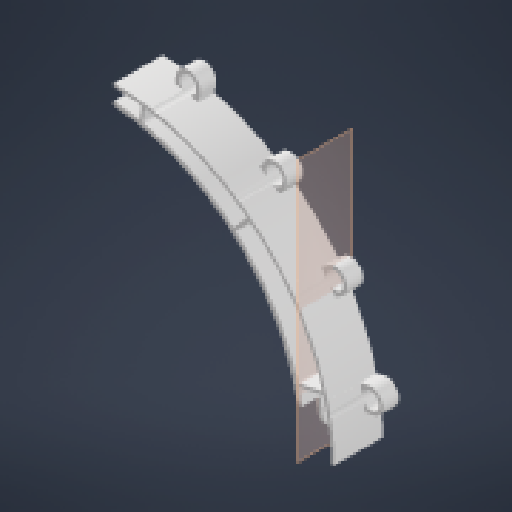
# Autodesk Inventor part: FilterSidewall
Saved by Autodesk Inventor 2026 (Build 300175050, 175E)
## iProperties
Created: 2026-05-05
Part Number: FilterSidewall
Material: Generic
Document SubType Name: Modeling
Designer: sniel
Density: 1 g/cm^3
Appearance: Default
Author: sniel
Autodesk Inventor part; units mm, degrees
ref_plane "YZ Plane" through (0, 0, 0) normal (1, 0, 0) x (0, 1, 0)
ref_plane "XZ Plane" through (0, 0, 0) normal (0, 1, 0) x (-1, 0, 0)
ref_plane "XY Plane" through (0, 0, 0) normal (0, 0, 1) x (1, 0, 0)
sketch "Sketch1" plane through (0, 0, 0) normal (0, 0, 1) x (1, 0, 0)
  circle A0 centre (-26.4627, 2.4988) radius 5.25
  circle A1 centre (-79.388, -19.4236) radius 5.25
  circle A2 centre (-138.7343, -109.7729) radius 5.25
  circle A3 centre (-116.8119, -56.8475) radius 5.25
  line L0 (-70.3746, -19.4683) -> (-73.0753, -15.2583)
  arc A4 (-73.0753, -15.2583) -> (-85.477, -23.6867) centre (-79.3881, -19.3078) ccw
  line L1 (-85.477, -23.6867) -> (-82.5566, -27.7475)
  arc A5 (-82.5566, -27.7475) -> (-108.3722, -53.5631) centre (0, -136.1197) ccw
  line L2 (-108.3722, -53.5631) -> (-112.433, -50.6428)
  arc A6 (-112.433, -50.6428) -> (-120.8615, -63.0445) centre (-116.8119, -56.7317) ccw
  line L3 (-120.8615, -63.0445) -> (-116.6514, -65.7451)
  arc A7 (-116.6514, -65.7451) -> (-132.2473, -103.397) centre (0, -136.1197) ccw
  line L4 (-132.2473, -103.397) -> (-137.134, -102.3297)
  arc A8 (-137.134, -102.3297) -> (-139.9435, -117.0589) centre (-138.7343, -109.657) ccw
  line L5 (-139.9435, -117.0589) -> (-135.0071, -117.8653)
  arc A9 (-135.0071, -117.8653) -> (-136.2355, -136.2355) centre (0, -136.1197) ccw
  line L6 (-136.2355, -136.2355) -> (-134.2355, -136.2355)
  arc A10 (0, -2) -> (-134.2355, -136.2355) centre (0, -136.2355) ccw
  line L7 (0, -2) -> (0, 0.1158)
  arc A11 (0, 0.1158) -> (-18.2544, -1.1127) centre (0, -136.1197) ccw
  line L8 (-18.2544, -1.1127) -> (-19.0608, 3.8237)
  arc A12 (-19.0608, 3.8237) -> (-33.79, 1.0142) centre (-26.4627, 2.6146) ccw
  line L9 (-33.79, 1.0142) -> (-32.7227, -3.8724)
  arc A13 (-32.7227, -3.8724) -> (-70.3746, -19.4683) centre (0, -136.1197) ccw
  circle A14 centre (138.7343, -109.7729) radius 5.25
  circle A15 centre (116.8119, -56.8475) radius 5.25
  circle A16 centre (26.4627, 2.4988) radius 5.25
  circle A17 centre (79.388, -19.4236) radius 5.25
  line L10 (116.6514, -65.7451) -> (120.8614, -63.0445)
  arc A18 (120.8614, -63.0445) -> (112.4329, -50.6428) centre (116.8119, -56.7317) ccw
  line L11 (112.4329, -50.6428) -> (108.3722, -53.5631)
  arc A19 (108.3722, -53.5631) -> (82.5566, -27.7475) centre (0, -136.1197) ccw
  line L12 (82.5566, -27.7475) -> (85.4769, -23.6867)
  arc A20 (85.4769, -23.6867) -> (73.0752, -15.2583) centre (79.388, -19.3078) ccw
  line L13 (73.0752, -15.2583) -> (70.3746, -19.4683)
  arc A21 (70.3746, -19.4683) -> (32.7226, -3.8724) centre (0, -136.1197) ccw
  line L14 (32.7226, -3.8724) -> (33.7899, 1.0142)
  arc A22 (33.7899, 1.0142) -> (19.0608, 3.8237) centre (26.4627, 2.6146) ccw
  line L15 (19.0608, 3.8237) -> (18.2544, -1.1127)
  arc A23 (18.2544, -1.1127) -> (0, 0.1158) centre (0, -136.1197) ccw
  line L16 (0, 0.1158) -> (0, -2)
  arc A24 (134.2355, -136.2355) -> (0, -2) centre (0, -136.2355) ccw
  line L17 (134.2355, -136.2355) -> (136.2355, -136.2355)
  arc A25 (136.2355, -136.2355) -> (135.007, -117.8653) centre (0, -136.1197) ccw
  line L18 (135.007, -117.8653) -> (139.9434, -117.0589)
  arc A26 (139.9434, -117.0589) -> (137.1339, -102.3297) centre (138.7343, -109.657) ccw
  line L19 (137.1339, -102.3297) -> (132.2473, -103.397)
  arc A27 (132.2473, -103.397) -> (116.6514, -65.7451) centre (0, -136.1197) ccw
  arc A28 (132.2355, -136.2355) -> (0, -4) centre (0, -136.2355) ccw projected
  line L20 (0, -4) -> (0, -31) projected
  arc A29 (105.2355, -136.2355) -> (0, -31) centre (0, -136.2355) ccw projected
  line L21 (105.2355, -136.2355) -> (132.2355, -136.2355) projected
  arc A30 (0, -4) -> (-132.2355, -136.2355) centre (0, -136.2355) ccw projected
  line L22 (-132.2355, -136.2355) -> (-105.2355, -136.2355) projected
  arc A31 (0, -31) -> (-105.2355, -136.2355) centre (0, -136.2355) ccw projected
  line L23 (0, -31) -> (0, -4) projected
  line L24 (105.2355, -136.2355) -> (115.2355, -136.2355)
  line L25 (132.2355, -136.2355) -> (118.2355, -136.2355)
  arc A32 (115.2355, -136.2355) -> (-134.2355, -136.2355) centre (-9.5, -136.2355) ccw
  arc A33 (118.2355, -136.2355) -> (-136.2355, -136.2355) centre (-9, -136.1273) ccw
  line L26 (17.9133, -3.2006) -> (16.6304, -11.5)
  line L27 (16.6304, -11.5) -> (18.5862, -11.9183)
  line L28 (18.5862, -11.9183) -> (19.8903, -3.4818)
  line L29 (73.9796, -39.6738) -> (82.5566, -30.3885)
  line L30 (73.9796, -39.6738) -> (75.4854, -40.99)
  line L31 (75.4854, -40.99) -> (84.1283, -31.6334)
  line L32 (113.8104, -102.8634) -> (114.3181, -104.7979)
  line L33 (114.3181, -104.7979) -> (129.6499, -101.4493)
  line L34 (113.8104, -102.8634) -> (129.1169, -99.5203)
  point P0 (-105.1806, -52.8316)
  dimension "d17" = 10
  dimension "d18" = 14
  dimension "d28" = 2
  dimension "d29" = 2
  dimension "d31" = 2
  constraints: 62 end point, 56 point on circle, 30 centre point, 3 parallel, 2 point on line, 2 tangent
  measures "d17" distance of L21.start L24.end
  measures "d18" distance of L21.end L25.end
  measures "d28" distance of L26.end L27.end
  measures "d29" distance of L29.start L30.end
  measures "d31" distance of L32.start L32.end
extrude "Extrusion1" add sketch "Sketch1" along normal blind 30 contours A2 A33 A9 L5 A8 L4 A7 L3 A6 L2 A5 L1 A4 L0 A13 L9 A12 L8 A11 L7 A10 | A2 A33 A10 L6 | A33 A30 A32 A10 | L7 A23 L15 A22 L14 A21 L13 A20 L12 A19 L11 A18 L10 A27 L19 A26 L18 A25 L17 A24 | A33 L20 A32 A30 | A24 L28 A28 L26 | A33 L27 L30 L32 L21 A32 L20 | A28 L28 A33 L26 | A33 L27 | A24 L31 A28 L29 | A28 L31 A33 L29 | A33 L30 | L32 A33 | A33 L34 A28 L33 | A24 L33 A28 L34
ref_plane "Work Plane1" through (115.2355, -136.2355, 0) normal (1, 0, 0) x (0, 0, 1)
sketch "Sketch2" plane through (115.2355, -136.2355, 0) normal (1, 0, 0) x (0, 0, 1)
  line L0 (0, 0) -> (30, 0) projected
  line L1 (30, 0) -> (30, -124.7355) projected
  line L2 (0, 0) -> (22, 0)
  line L3 (0, -4.5) -> (30, -4.5)
  line L4 (0, -4.5) -> (22, -4.5)
  line L5 (11, -4.5) -> (11, -12)
  circle A0 centre (11, -12) radius 7.5
  line L6 (18.5, -12) -> (18.5, -22)
  line L7 (3.5, -12) -> (3.5, -22)
  line L8 (3.5, -22) -> (0, -22)
  line L9 (18.5, -22) -> (30, -22)
  line L10 (30, 0) -> (30, -22)
  line L11 (0, -4.5) -> (30, -4.5)
  line L12 (30, -4.5) -> (30, 0)
  line L13 (30, 0) -> (0, 0)
  line L14 (0, 0) -> (0, -4.5)
  line L15 (0, -31.4376) -> (0, 0) projected
  line L16 (0, -22) -> (0, 0)
  point P0 (0, -136.2355)
  point P1 (30, -17.5)
  point P2 (30, -22)
  dimension "d21" = 22
  dimension "d35" = 22
  dimension "d36" = 7.5
  dimension "d37" = 10
  dimension "d38" = 22
  constraints: 28 end point, 5 point on line, 4 vertical, 3 point on circle, 2 parallel, 1 centre point, 1 coincident, 1 horizontal, 1 midpoint, 1 perpendicular, 1 tangent
  measures "d21" distance of L0.start L2.end
  measures "d35" distance of L3.start L4.end
  measures "d36" distance of L5.start L5.end
  measures "d37" distance of L6.start L6.end
  measures "d38" distance of L0.end L10.end
extrude "Extrusion2" cut sketch "Sketch2" along normal mid plane 13.75 contours L0 L1 L3 L14 | L3 A0 L7 L8 L15 | L3 L1 L9 L6 A0
sketch "Sketch3" plane through (0, 0, 30) normal (0, 0, 1) x (1, 0, 0)
  line L0 (114.0018, -118.7355) -> (117.0413, -118.7355)
  arc A0 (117.0413, -118.7355) -> (-105.1806, -52.8316) centre (-9, -136.1273) ccw
  arc A1 (134.2355, -136.2355) -> (-105.1806, -52.8316) centre (0, -136.2355) ccw
  line L1 (134.2355, -136.2355) -> (136.2355, -136.2355)
  arc A2 (136.2355, -136.2355) -> (135.007, -117.8653) centre (0, -136.1197) ccw
  line L2 (135.007, -117.8653) -> (139.9434, -117.0589)
  arc A3 (139.9434, -117.0589) -> (137.1339, -102.3297) centre (138.7343, -109.657) ccw
  line L3 (137.1339, -102.3297) -> (132.2473, -103.397)
  arc A4 (132.2473, -103.397) -> (116.6514, -65.7451) centre (0, -136.1197) ccw
  line L4 (116.6514, -65.7451) -> (120.8614, -63.0445)
  arc A5 (120.8614, -63.0445) -> (112.4329, -50.6428) centre (116.8119, -56.7317) ccw
  line L5 (112.4329, -50.6428) -> (108.3722, -53.5631)
  arc A6 (108.3722, -53.5631) -> (82.5566, -27.7475) centre (0, -136.1197) ccw
  line L6 (82.5566, -27.7475) -> (85.4769, -23.6867)
  arc A7 (85.4769, -23.6867) -> (73.0752, -15.2583) centre (79.388, -19.3078) ccw
  line L7 (73.0752, -15.2583) -> (70.3746, -19.4683)
  arc A8 (70.3746, -19.4683) -> (32.7226, -3.8724) centre (0, -136.1197) ccw
  line L8 (32.7226, -3.8724) -> (33.7899, 1.0142)
  arc A9 (33.7899, 1.0142) -> (19.0608, 3.8237) centre (26.4627, 2.6146) ccw
  line L9 (19.0608, 3.8237) -> (18.2544, -1.1127)
  arc A10 (18.2544, -1.1127) -> (-18.2544, -1.1127) centre (0, -136.1201) ccw
  line L10 (-18.2544, -1.1127) -> (-19.0608, 3.8237)
  arc A11 (-19.0608, 3.8237) -> (-33.79, 1.0142) centre (-26.4627, 2.6146) ccw
  line L11 (-33.79, 1.0142) -> (-32.7227, -3.8724)
  arc A12 (-32.7227, -3.8724) -> (-70.3746, -19.4683) centre (0, -136.1197) ccw
  line L12 (-70.3746, -19.4683) -> (-73.0753, -15.2583)
  arc A13 (-73.0753, -15.2583) -> (-85.477, -23.6867) centre (-79.3881, -19.3078) ccw
  line L13 (-85.477, -23.6867) -> (-82.5566, -27.7475)
  arc A14 (-82.5566, -27.7475) -> (-108.3722, -53.5631) centre (0, -136.1197) ccw
  line L14 (-108.3722, -53.5631) -> (-112.433, -50.6428)
  arc A15 (-112.433, -50.6428) -> (-120.8615, -63.0445) centre (-116.8119, -56.7317) ccw
  line L15 (-120.8615, -63.0445) -> (-116.6514, -65.7451)
  arc A16 (-116.6514, -65.7451) -> (-132.2473, -103.397) centre (0, -136.1197) ccw
  line L16 (-132.2473, -103.397) -> (-137.134, -102.3297)
  arc A17 (-137.134, -102.3297) -> (-139.9435, -117.0589) centre (-138.7343, -109.657) ccw
  line L17 (-139.9435, -117.0589) -> (-135.0071, -117.8653)
  arc A18 (-135.0071, -117.8653) -> (-136.2355, -136.2355) centre (0, -136.1197) ccw
  line L18 (-136.2355, -136.2355) -> (-134.2355, -136.2355)
  arc A19 (114.0018, -118.7355) -> (-134.2355, -136.2355) centre (-9.5, -136.2355) ccw
  circle A20 centre (138.7343, -109.7729) radius 5.25
  circle A21 centre (116.8119, -56.8475) radius 5.25
  circle A22 centre (26.4627, 2.4988) radius 5.25
  circle A23 centre (79.388, -19.4236) radius 5.25
  circle A24 centre (-138.7343, -109.7729) radius 5.25
  circle A25 centre (-116.8119, -56.8475) radius 5.25
  circle A26 centre (-79.388, -19.4236) radius 5.25
  circle A27 centre (-26.4627, 2.4988) radius 5.25
  line L19 (0, 0.1158) -> (0, -11.8623)
  point P0 (0, -9.2105)
  point P1 (0, -2)
  constraints: 56 centre point, 42 point on circle, 40 end point, 1 vertical
extrude "Extrusion3" cut sketch "Sketch3" against normal blind 31 contours A19 L18 A18 L17 A17 L16 A16 L15 A15 L14 A14 L13 A13 L12 A12 L11 A11 L10 A10 L19 A1 A0
fillet "Fillet1" radius 1 18 edges at (0, 0.1158, 15) (0, -2, 15) (0, -9.2105, 15) (0, -11.8623, 15) (17.9133, -3.2006, 15) (19.8903, -3.4818, 15) (16.6304, -11.5, 15) (18.5862, -11.9183, 15) (73.9796, -39.6738, 15) (75.4854, -40.99, 15) (84.1283, -31.6334, 15) (82.5566, -30.3885, 15) (129.6499, -101.4493, 15) (114.3181, -104.7979, 15) (113.8104, -102.8634, 15) (129.1169, -99.5203, 15) (134.2355, -136.2355, 15) (136.2355, -136.2355, 15)
sketch "Sketch4" plane through (0, 0, 30) normal (0, 0, 1) x (1, 0, 0)
  circle A0 centre (138.7343, -109.7729) radius 5.25 projected
  circle A1 centre (116.8119, -56.8475) radius 5.25 projected
  circle A2 centre (26.4627, 2.4988) radius 5.25 projected
  circle A3 centre (79.388, -19.4236) radius 5.25 projected
  arc A4 (81.6899, -29.7183) -> (20.8815, -3.6341) centre (0, -136.2355) ccw projected
  arc A5 (81.816, -31.1903) -> (81.6899, -29.7183) centre (81.0814, -30.5118) ccw projected
  line L0 (81.816, -31.1903) -> (74.6321, -38.9674) projected
  arc A6 (73.2511, -39.0518) -> (74.6321, -38.9674) centre (73.8975, -38.2889) ccw projected
  arc A7 (73.2511, -39.0518) -> (19.4931, -12.1232) centre (-9, -136.1273) ccw projected
  arc A8 (18.7288, -10.9958) -> (19.4931, -12.1232) centre (19.717, -11.1486) ccw projected
  line L1 (18.7288, -10.9958) -> (19.7377, -4.4692) projected
  arc A9 (20.8815, -3.6341) -> (19.7377, -4.4692) centre (20.7259, -4.6219) ccw projected
  arc A10 (113.5601, -101.9527) -> (76.2393, -41.6649) centre (-9, -136.1273) ccw projected
  arc A11 (76.1746, -40.2439) -> (76.2393, -41.6649) centre (76.9092, -40.9225) ccw projected
  line L2 (76.1746, -40.2439) -> (83.4925, -32.3218) projected
  arc A12 (84.8592, -32.2255) -> (83.4925, -32.3218) centre (84.227, -33.0003) ccw projected
  arc A13 (128.8195, -98.4901) -> (84.8592, -32.2255) centre (0, -136.2355) ccw projected
  arc A14 (128.0732, -99.7482) -> (128.8195, -98.4901) centre (127.8598, -98.7713) ccw projected
  line L3 (128.0732, -99.7482) -> (114.7368, -102.6611) projected
  arc A15 (113.5601, -101.9527) -> (114.7368, -102.6611) centre (114.5234, -101.6841) ccw projected
  arc A16 (135.2326, -136.2355) -> (136.2326, -135.229) centre (135.2326, -135.2355) ccw projected
  arc A17 (136.2326, -135.229) -> (135.007, -117.8653) centre (0, -136.1197) ccw projected
  line L4 (135.007, -117.8653) -> (139.9434, -117.0589) projected
  arc A18 (139.9434, -117.0589) -> (137.1339, -102.3297) centre (138.7343, -109.657) ccw projected
  line L5 (137.1339, -102.3297) -> (132.2473, -103.397) projected
  arc A19 (132.2473, -103.397) -> (116.6514, -65.7451) centre (0, -136.1197) ccw projected
  line L6 (116.6514, -65.7451) -> (120.8614, -63.0445) projected
  arc A20 (120.8614, -63.0445) -> (112.4329, -50.6428) centre (116.8119, -56.7317) ccw projected
  line L7 (112.4329, -50.6428) -> (108.3722, -53.5631) projected
  arc A21 (108.3722, -53.5631) -> (82.5566, -27.7475) centre (0, -136.1197) ccw projected
  line L8 (82.5566, -27.7475) -> (85.4769, -23.6867) projected
  arc A22 (85.4769, -23.6867) -> (73.0752, -15.2583) centre (79.388, -19.3078) ccw projected
  line L9 (73.0752, -15.2583) -> (70.3746, -19.4683) projected
  arc A23 (70.3746, -19.4683) -> (32.7226, -3.8724) centre (0, -136.1197) ccw projected
  line L10 (32.7226, -3.8724) -> (33.7899, 1.0142) projected
  arc A24 (33.7899, 1.0142) -> (19.0608, 3.8237) centre (26.4627, 2.6146) ccw projected
  line L11 (19.0608, 3.8237) -> (18.2544, -1.1127) projected
  arc A25 (18.2544, -1.1127) -> (1.0074, 0.1121) centre (0, -136.1201) ccw projected
  arc A26 (1.0074, 0.1121) -> (0, -0.8879) centre (1, -0.8879) ccw projected
  line L12 (0, -0.8879) -> (0, -1.0037) projected
  arc A27 (0, -1.0037) -> (0.9926, -2.0037) centre (1, -1.0037) ccw projected
  arc A28 (16.8945, -3.0674) -> (0.9926, -2.0037) centre (0, -136.2355) ccw projected
  arc A29 (17.7569, -4.2122) -> (16.8945, -3.0674) centre (16.7687, -4.0594) ccw projected
  line L13 (17.7569, -4.2122) -> (16.7902, -10.4659) projected
  arc A30 (15.6086, -11.2942) -> (16.7902, -10.4659) centre (15.802, -10.3131) ccw projected
  arc A31 (15.6086, -11.2942) -> (1.0792, -9.2916) centre (-9, -136.1273) ccw projected
  arc A32 (1.0792, -9.2916) -> (0, -10.2885) centre (1, -10.2885) ccw projected
  line L14 (0, -10.2885) -> (0, -10.9392) projected
  arc A33 (0, -10.9392) -> (0.9165, -11.9357) centre (1, -10.9392) ccw projected
  arc A34 (113.2801, -114.2355) -> (0.9165, -11.9357) centre (-9.5, -136.2355) ccw projected
  arc A35 (116.3381, -114.2355) -> (114.5668, -105.7934) centre (-9, -136.1273) ccw projected
  arc A36 (115.3246, -104.5781) -> (114.5668, -105.7934) centre (115.5379, -105.555) ccw projected
  line L15 (115.3246, -104.5781) -> (128.7145, -101.6535) projected
  arc A37 (129.8956, -102.3783) -> (128.7145, -101.6535) centre (128.9279, -102.6305) ccw projected
  arc A38 (134.2319, -135.2429) -> (129.8956, -102.3783) centre (0, -136.2355) ccw projected
  arc A39 (134.2319, -135.2429) -> (135.2318, -136.2355) centre (135.2318, -135.2355) ccw projected
  line L16 (135.2318, -136.2355) -> (135.2326, -136.2355) projected
  circle A40 centre (0, -136.2355) radius 136.3503
  line L17 (113.2801, -114.2355) -> (116.3381, -114.2355) projected
  point P0 (0, 0)
  point P1 (132.3323, -103.3785)
  point P2 (133.5688, -108.8349)
  point P3 (134.2767, -112.5464)
  point P4 (135.105, -117.8493)
  point P5 (108.4084, -53.5371)
  point P6 (111.6987, -58.0383)
  point P7 (113.8226, -61.1634)
  point P8 (116.6976, -65.7155)
  point P9 (70.383, -19.4552)
  point P10 (75.0722, -22.4129)
  point P11 (78.1972, -24.5368)
  point P12 (82.5698, -27.7291)
  point P13 (23.6891, -1.9588)
  point P14 (27.4007, -2.6668)
  point P15 (32.7231, -3.8701)
  constraints: 1 coincident, 3 other
extrude "Extrusion4" cut sketch "Sketch4" against normal blind 20 contours A0 A40 L5 A18 L4 | A40 A1 L7 A20 L6 | L11 A24 L10 A40 A2 | A40 A3 L9 A22 L8
body "Solid1"
